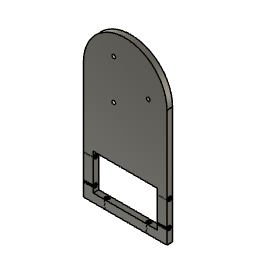
Viewing_plate (Autodesk Fusion 360 design; units mm, degrees)
Autodesk Fusion 360 part; units mm, degrees
sketch "Sketch1" plane through (0, 0, 0) normal (0, 1, 0) x (1, 0, 0)
  circle A0 centre (0, 0) radius 20.05 construction
  line L0 (-30, 0) -> (30, 0) construction
  line L1 (30, 0) -> (30, 100)
  line L2 (30, 100) -> (-30, 100)
  line L3 (-30, 100) -> (-30, 0)
  circle A1 centre (0, 0) radius 30 construction
  circle A2 centre (0, 0) radius 30
  dimension "d1" = 40.1
  dimension "d6" = 100
  dimension "d9" = 60
  dimension "d10" = 60
  dimension "d11" = 30
  constraint coincident A0.centre A1.centre
  constraint horizontal L0
  constraint perpendicular L0 L1
  constraint perpendicular L1 L2
  constraint perpendicular L0 L3
  constraint concentric A0 A1
  constraint coincident L0.end A1
  constraint tangent L1 A1
  constraint concentric A0 A2
  measures "d1" diameter of A0
  measures "d6" distance of L0.end L1.end
  measures "d9" distance of L1.end L2.end
  measures "d10" diameter of A2
  measures "d11" distance of L1 A0.centre
extrude "Extrude1" add sketch "Sketch1" along normal blind 4
sketch "Sketch2" plane through (0, 0, 0) normal (0, -1, 0) x (1, 0, 0)
  line L0 (-30, 0) -> (-30, -100)
  line L1 (-30, -100) -> (30, -100)
  line L2 (30, -100) -> (30, 0)
  arc A0 (30, 0) -> (-30, 0) centre (0, 0) ccw
  line L3 (-23, -78.04) -> (23, -78.04)
  line L4 (23, -78.04) -> (23, -52.04)
  line L5 (23, -52.04) -> (-23, -52.04)
  line L6 (-23, -52.04) -> (-23, -78.04)
  line L7 (-30, -100) -> (30, -100)
  line L8 (30, -100) -> (30, -84)
  line L9 (30, -84) -> (-30, -84)
  line L10 (-30, -84) -> (-30, -100)
  dimension "d7" = 21.96
  dimension "d8" = 26
  dimension "d12" = 46
  dimension "d13" = 23
  dimension "d14" = 16
  constraint horizontal L3
  constraint vertical L4
  constraint horizontal L5
  constraint vertical L6
  constraint horizontal L7
  constraint vertical L8
  constraint horizontal L9
  constraint vertical L10
  constraint coincident L0.end L1.start
  measures "d7" distance of L1 L3
  measures "d8" distance of L3.end L4.end
  measures "d12" distance of L4.end L5.end
  measures "d13" distance of A0.centre L4
  measures "d14" distance of L0.end L9.end
extrude "Extrude2" cut sketch "Sketch2" against normal blind 15 contours L0 L1 L2 L7 L8 L9 L10 | L3 L4 L5 L6
sketch "Sketch3" plane through (-23, 0, 0) normal (1, 0, 0) x (0, 1, 0)
  line L0 (0, -52.04) -> (0, -78.04)
  line L1 (0, -78.04) -> (4, -78.04)
  line L2 (4, -52.04) -> (0, -52.04)
  line L3 (2, -78.04) -> (2, -52.04) construction
  line L4 (5.0337, -65.1397) -> (0, -65.04) construction
  circle A0 centre (2, -56.0779) radius 1.5
  circle A1 centre (1.6435, -74.0743) radius 1.5
  line L5 (4, -78.04) -> (4, -52.04)
  dimension "d15" = 3
  dimension "d16" = 9
  constraint midpoint L1 L3.start
  constraint midpoint L2 L3.end
  constraint midpoint L0 L4.end
  constraint coincident L3 A0.centre
  constraint symmetric L4 A0 A1
  measures "d15" diameter of A0
  measures "d16" distance of L4 A0.centre
hole "Hole1" at (-23, 2, -56.0779) at (-23, 1.6435, -74.0743) direction (-1, 0, 0) diameter 3 depth 14 tip angle 118
thread "Thread1" "ISO Metric profile 3.0 M3x0.5 6H" major diameter 3.086 minor diameter 2.529 pitch 0.5 angle 60 modelled right hand crest width 0.1368 on face at (-27.6667, 3.3348, -55.3935) crest through (-23.125, 3.2645, -56.0779) on face at (-25.3333, 1.7182, -75.5725) crest through (-23.125, 2.908, -74.0743)
sketch "Sketch4" plane through (23, 0, 0) normal (-1, 0, 0) x (0, -1, 0)
  line L0 (0, -78.04) -> (0, -52.04)
  line L1 (0, -52.04) -> (-4, -52.04)
  line L2 (-4, -78.04) -> (0, -78.04)
  line L3 (-2, -78.04) -> (-2, -52.04) construction
  line L4 (-5.0337, -65.1397) -> (0, -65.04) construction
  circle A0 centre (-2, -56.0779) radius 1.5
  circle A1 centre (-1.6435, -74.0743) radius 1.5
  line L5 (-4, -52.04) -> (-4, -78.04)
  dimension "d20" = 3
  dimension "d21" = 9
  constraint midpoint L2 L3.start
  constraint midpoint L1 L3.end
  constraint midpoint L0 L4.end
  constraint coincident L3 A0.centre
  constraint symmetric L4 A0 A1
  measures "d20" diameter of A0
  measures "d21" distance of L4 A0.centre
hole "Hole2" at (23, 2, -56.0779) at (23, 1.6435, -74.0743) direction (1, 0, 0) diameter 3 depth 14 tip angle 118
thread "Thread2" "ISO Metric profile 3.0 M3x0.5 6H" major diameter 3.086 minor diameter 2.529 pitch 0.5 angle 60 modelled right hand crest width 0.1368 on face at (27.6667, 3.3348, -56.7622) crest through (23.125, 0.7355, -56.0779) on face at (25.3333, 1.7182, -72.5762) crest through (23.125, 0.379, -74.0743)
sketch "Sketch5" plane through (0, 0, -78.04) normal (0, 0, 1) x (-1, 0, 0)
  line L0 (23, 0) -> (-23, 0)
  line L1 (-23, 0) -> (-23, -4)
  line L2 (23, -4) -> (23, 0)
  line L3 (0, -4) -> (0, 0) construction
  line L4 (23, -2) -> (-23, -2) construction
  circle A0 centre (-15, -2) radius 1.5
  circle A1 centre (15, -2) radius 1.5
  line L5 (-23, -4) -> (23, -4)
  dimension "d25" = 3
  dimension "d26" = 15
  constraint coincident L3.end origin
  constraint midpoint L2 L4.start
  constraint midpoint L1 L4.end
  constraint coincident L4 A0.centre
  constraint symmetric L3 A0 A1
  constraint midpoint L3.start L5
  measures "d25" diameter of A0
  measures "d26" distance of L3 A0.centre
hole "Hole3" at (-15, 2, -78.04) at (15, 2, -78.04) direction (0, 0, -1) diameter 3 depth 14 tip angle 118
thread "Thread3" "ISO Metric profile 3.0 M3x0.5 6H" major diameter 3.086 minor diameter 2.529 pitch 0.5 angle 60 modelled right hand crest width 0.1368 on face at (-14.9252, 0.5019, -80.0267) crest through (-13.7355, 2, -78.165) on face at (15.0748, 0.5019, -80.0267) crest through (16.2645, 2, -78.165)
sketch "Sketch6" plane through (0, 0, 0) normal (0, -1, 0) x (1, 0, 0)
  line L0 (-30, -84) -> (30, -84)
  line L1 (30, -84) -> (30, 0)
  arc A0 (30, 0) -> (-30, 0) centre (0, 0) ccw
  line L2 (-30, 0) -> (-30, -84)
  line L3 (23, -78.04) -> (-23, -78.04)
  line L4 (-23, -78.04) -> (-23, -52.04)
  line L5 (-23, -52.04) -> (23, -52.04)
  line L6 (23, -52.04) -> (23, -78.04)
  line L7 (0, 0) -> (0, 30) construction
  line L8 (0, 0) -> (-8.255, 14.2981) construction
  circle A1 centre (-8.255, 14.2981) radius 1.5
  circle A2 centre (-8.255, -14.2981) radius 1.5
  circle A3 centre (16.51, 0) radius 1.5
  dimension "d30" = 150
  dimension "d31" = 16.51
  dimension "d32" = 3
  dimension "d34" = 360
  constraint coincident A0.centre L7.start
  constraint midpoint A0 L7.end
  constraint coincident L8.end A1.centre
  measures "d30" angle of L7 L8
  measures "d31" distance of A0.centre L8.end
  measures "d32" diameter of A1
hole "Hole4" at (-8.255, 0, 14.2981) at (16.51, 0, 0) at (-8.255, 0, -14.2981) direction (0, 1, 0) diameter 3 depth 16 tip angle 118
thread "Thread4" "ISO Metric profile 3.0 M3x0.5 6H" major diameter 3.086 minor diameter 2.529 pitch 0.5 angle 60 resizes the face on face at (-8.1056, 2.6667, -15.7906) on face at (-8.1056, 2.6667, 12.8055) on face at (16.6594, 2.6667, -1.4925)
